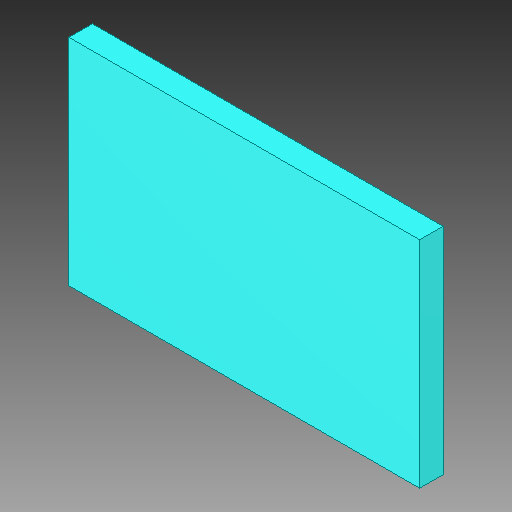
# Autodesk Inventor part: W237-103
Saved by Autodesk Inventor 2019 (Build 230136000, 136)
## iProperties
Created: 2019-10-02
Part Number: W237-103
Material: Generic
Document SubType Name: Modeling
Designer: rybit
Density: 1 g/cm^3
Appearance: W237-103, W237-103
Author: rybit
Autodesk Inventor part; units mm, degrees
ref_plane "YZ Plane" through (0, 0, 0) normal (1, 0, 0) x (0, 1, 0)
ref_plane "XZ Plane" through (0, 0, 0) normal (0, 1, 0) x (-1, 0, 0)
ref_plane "XY Plane" through (0, 0, 0) normal (0, 0, 1) x (1, 0, 0)
sketch "W237-103, W237-103_27" plane through (0, 0, 0) normal (0, 0, 1) x (1, 0, 0)
  line L0 (-7.489, 3.714) -> (7.497, 3.714)
  line L1 (7.497, 3.714) -> (7.497, -5.481)
  line L2 (7.497, -5.481) -> (-7.489, -5.481)
  line L3 (-7.489, -5.481) -> (-7.489, 3.714)
  constraints: 8 end point
extrude "Extrusion1" add sketch "W237-103, W237-103_27" along normal blind 1
body "Solid1"
